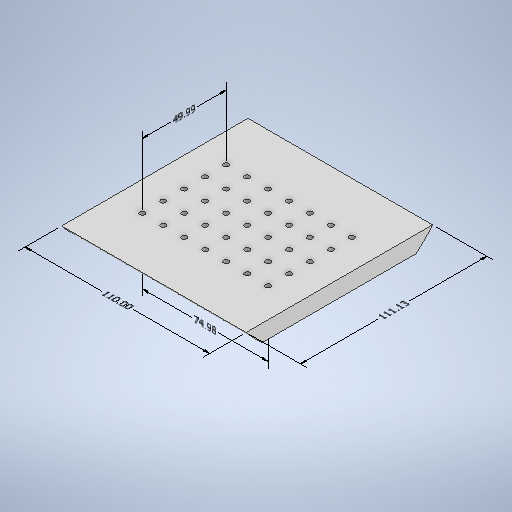
# Autodesk Inventor part: Base
Saved by Autodesk Inventor 2025.3 (Build 293356000, 356)
## iProperties
Created: 2025-05-16
Part Number: Base
Material: Generic
Document SubType Name: Modeling
Designer: Verðandi
Density: 1 g/cm^3
Appearance: Default
Author: Verðandi
Autodesk Inventor part; units mm, degrees
ref_plane "YZ Plane" through (0, 0, 0) normal (1, 0, 0) x (0, 1, 0)
ref_plane "XZ Plane" through (0, 0, 0) normal (0, 1, 0) x (-1, 0, 0)
ref_plane "XY Plane" through (0, 0, 0) normal (0, 0, 1) x (1, 0, 0)
sketch "Sketch1" plane through (0, 0, 0) normal (1, 0, 0) x (0, 1, 0)
  circle A0 centre (0, 0) radius 71
  dimension "d0" = 142
  constraints: 1 centre point, 1 coincident
  measures "d0" diameter of A0
extrude "Extrusion1" add sketch "Sketch1" along normal blind 110
sketch "Sketch2" plane through (110, 0, 0) normal (1, 0, 0) x (0, 0, -1)
  line L0 (0, 0) -> (0, -44.2)
  circle A0 centre (0, 0) radius 71 projected
  line L1 (-55.564, -44.2) -> (55.564, -44.2)
  dimension "d3" = 44.2
  constraints: 4 end point, 2 point on circle, 1 horizontal, 1 vertical
  measures "d3" distance of L0.start L0.end
extrude "Extrusion2" cut sketch "Sketch2" against normal blind 150 contours A0 L1 picked at (-0.2063, 32.437)
sketch "Sketch3" plane through (110, 0, 0) normal (1, 0, 0) x (0, 0, -1)
  line L0 (0, 0) -> (0, -54.2)
  arc A0 (-55.564, -44.2) -> (55.564, -44.2) centre (0, 0) ccw projected
  line L1 (-45.8624, -54.2) -> (45.8624, -54.2)
  dimension "d6" = 54.2
  constraints: 4 end point, 2 point on circle, 1 horizontal, 1 vertical
  measures "d6" distance of L0.start L0.end
extrude "Extrusion3" cut sketch "Sketch3" against normal blind 150
sketch "Sketch7" plane through (110, -44.2, 55.564) normal (0, 1, 0) x (1, 0, 0)
  line L0 (-110, 0) -> (-110, 9.7016) projected
  line L1 (-110, 0) -> (-55, 0)
  line L2 (0, 0) -> (-110, 0) projected
  line L3 (-110, 111.128) -> (0, 111.128) projected
  line L4 (-55, 0) -> (-55, 55.64)
  circle A0 centre (-55, 55.64) radius 1.5
  point P0 (-110, 55.564)
  dimension "d71" = 55
  dimension "d72" = 111.128
  dimension "d73" = 55.64
  dimension "d75" = 3
  constraints: 4 end point, 1 centre point, 1 coincident, 1 midpoint, 1 vertical
  measures "d71" distance of L0.start L1.end
  measures "d72" distance between parallel lines of L2 L3
  measures "d73" distance of L1.end L4.end
  measures "d75" diameter of A0
extrude "Extrusion5" cut sketch "Sketch7" against normal blind 10
pattern_linear "Rectangular Pattern1" count 7 spacing 12.4968 along (-1, 0, 0) count 5 spacing 12.4968 along (0, 0, -1) of "Extrusion2", "Extrusion5" first direction both ways yes second direction both ways yes
body "Solid1"
